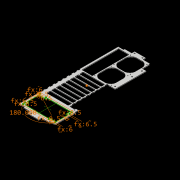
# Autodesk Inventor part: backpanel
Saved by Autodesk Inventor 2018 (Build 220112000, 112)
## iProperties
Created: 2019-10-14
Part Number: backpanel
Material: アルミニウム 6061
Document SubType Name: Modeling
Designer: gisen
Density: 2.7 g/cm^3
Appearance: アルミニウム - フラット
Author: gisen
Autodesk Inventor part; units mm, degrees
ref_plane "YZ Plane" through (0, 0, 0) normal (1, 0, 0) x (0, 1, 0)
ref_plane "XZ Plane" through (0, 0, 0) normal (0, 1, 0) x (-1, 0, 0)
ref_plane "XY Plane" through (0, 0, 0) normal (0, 0, 1) x (1, 0, 0)
sketch "スケッチ1" plane through (0, 0, 0) normal (0, 0, 1) x (1, 0, 0)
  line L0 (-55, -215) -> (55, -215) construction
  line L1 (55, -215) -> (55, 215) construction
  line L2 (55, 215) -> (-55, 215) construction
  line L3 (-55, 215) -> (-55, -215) construction
  line L4 (-55, -215) -> (55, 215) construction
  line L5 (55, -215) -> (-55, 215) construction
  line L6 (-75, 215) -> (-55, 215)
  line L7 (-55, 215) -> (-55, 232.5)
  line L8 (-55, 232.5) -> (55, 232.5)
  line L9 (55, 232.5) -> (55, 215)
  line L10 (55, 215) -> (75, 215)
  line L11 (75, 215) -> (75, -215)
  line L12 (75, -215) -> (55, -215)
  line L13 (55, -215) -> (55, -232.5)
  line L14 (55, -232.5) -> (-55, -232.5)
  line L15 (-55, -232.5) -> (-55, -215)
  line L16 (-55, -215) -> (-75, -215)
  line L17 (-75, -215) -> (-75, 215)
  line L18 (-65, 225) -> (65, 225) construction
  line L19 (65, 225) -> (65, -225) construction
  line L20 (65, -225) -> (-65, -225) construction
  line L21 (-65, -225) -> (-65, 225) construction
  circle A0 centre (-45, 225) radius 2.25
  circle A1 centre (-65, 205) radius 2.25
  line L22 (0, 0) -> (0, 232.5) construction
  line L23 (0, 0) -> (-75, 0) construction
  circle A2 centre (45, 225) radius 2.25
  circle A3 centre (65, 205) radius 2.25
  circle A4 centre (-45, -225) radius 2.25
  circle A5 centre (-65, -205) radius 2.25
  circle A6 centre (45, -225) radius 2.25
  circle A7 centre (65, -205) radius 2.25
  dimension "d0" = 110
  dimension "d1" = 430
  dimension "d2" = 17.5
  dimension "d3" = 17.5
  dimension "d4" = 20
  dimension "d5" = 20
  dimension "d6" = 10
  dimension "d7" = 10
  dimension "d8" = 10
  dimension "d9" = 10
  dimension "d10" = 4.5
  dimension "d11" = 10
  dimension "d12" = 10
  constraints: 48 end point, 8 centre point, 6 perpendicular, 6 point on line, 6 symmetric about line, 5 parallel, 4 midpoint, 4 vertical, 3 horizontal, 1 equal radius, 6 other
  measures "d0" distance of L2.end L1.end
  measures "d1" distance of L1.end L0.end
  measures "d2" distance of L8.end L1.end
  measures "d3" distance of L0.end L13.end
  measures "d4" distance of L1.end L10.end
  measures "d5" distance of L6.start L2.end
  measures "d6" distance between parallel lines of L2 L18
  measures "d7" distance between parallel lines of L3 L21
  measures "d8" distance between parallel lines of L0 L20
  measures "d9" distance between parallel lines of L1 L19
  measures "d10" diameter of A0
  measures "d11" distance from line of L7 A0.centre
  measures "d12" distance from line of A1.centre L6
extrude "押し出し1" add sketch "スケッチ1" along normal blind 3 contours L6 L7 L8 L9 L10 L11 L12 L13 L14 L15 L16 L17 | A1 | A5 | A7
sketch "スケッチ2" plane through (0, 0, 3) normal (0, 0, 1) x (1, 0, 0)
  line L0 (-68.0594, 208.0035) -> (-25.8794, 208.0035) construction
  line L1 (-69.2594, 50.3235) -> (-69.2594, 206.8035) construction
  line L2 (-25.8794, 49.1235) -> (-68.0594, 49.1235) construction
  line L3 (-24.6794, 206.8035) -> (-24.6794, 50.3235) construction
  line L4 (-24.6794, 49.1235) -> (-69.2594, 49.1235) construction
  line L5 (-69.2594, 49.1235) -> (-69.2594, 208.0035) construction
  line L6 (-69.2594, 208.0035) -> (-24.6794, 208.0035) construction
  line L7 (-24.6794, 208.0035) -> (-24.6794, 49.1235) construction
  line L8 (-24.6794, 49.1235) -> (-69.2594, 208.0035) construction
  line L9 (-69.2594, 49.1235) -> (-24.6794, 208.0035) construction
  line L10 (-69.3194, 49.0635) -> (-24.6194, 49.0635)
  line L11 (-24.6194, 49.0635) -> (-24.6194, 208.0635)
  line L12 (-24.6194, 208.0635) -> (-69.3194, 208.0635)
  line L13 (-69.3194, 208.0635) -> (-69.3194, 49.0635)
  line L14 (-69.3194, 49.0635) -> (-24.6194, 208.0635) construction
  line L15 (-24.6194, 49.0635) -> (-69.3194, 208.0635) construction
  point P0 (0, 0)
  point P1 (-46.9694, 128.5635)
  point P2 (-46.9694, 208.0035)
  point P3 (-69.2594, 128.5635)
  dimension "d16" = 44.7
  dimension "d17" = 159
  constraints: 24 end point, 8 midpoint, 4 parallel, 2 horizontal, 2 perpendicular
  measures "d16" distance of L12.end L11.end
  measures "d17" distance of L11.end L10.end
extrude "押し出し2" cut sketch "スケッチ2" against normal blind 3
sketch "スケッチ3" plane through (0, 0, 3) normal (0, 0, 1) x (1, 0, 0)
  line L0 (-70.0884, -112.7392) -> (-77.313, -112.7392) construction
  line L1 (-77.313, -102.4522) -> (-70.0884, -102.4522) construction
  line L2 (-70.0884, -92.3938) -> (-77.313, -92.3938) construction
  line L3 (-77.313, -82.1068) -> (-70.0884, -82.1068) construction
  line L4 (-70.0884, -71.7392) -> (-77.313, -71.7392) construction
  line L5 (-77.313, -61.4522) -> (-70.0884, -61.4522) construction
  line L6 (-70.0884, -51.3938) -> (-77.313, -51.3938) construction
  line L7 (-77.313, -41.1068) -> (-70.0884, -41.1068) construction
  line L8 (-70.0884, -30.7392) -> (-77.313, -30.7392) construction
  line L9 (-77.313, -20.4522) -> (-70.0884, -20.4522) construction
  line L10 (-70.0884, -10.3938) -> (-77.313, -10.3938) construction
  line L11 (-77.313, -0.1068) -> (-70.0884, -0.1068) construction
  line L12 (-70.0884, 10.2608) -> (-77.313, 10.2608) construction
  line L13 (-77.313, 20.5478) -> (-70.0884, 20.5478) construction
  line L14 (-70.0884, 30.6062) -> (-77.313, 30.6062) construction
  line L15 (-77.313, 40.8932) -> (-70.0884, 40.8932) construction
  line L16 (-75, 215) -> (-75, -215) projected
  line L17 (-75, 46.0635) -> (-78, 46.0635)
  line L18 (-78, 46.0635) -> (-78, 215)
  line L19 (-78, 215) -> (-75, 215)
  line L20 (-75, 215) -> (-75, 46.0635)
  line L21 (-24.6194, 49.0635) -> (-69.3194, 49.0635) projected
  line L22 (-75, -112.7392) -> (-78, -112.7392)
  line L23 (-78, -112.7392) -> (-78, -102.4522)
  line L24 (-78, -102.4522) -> (-75, -102.4522)
  line L25 (-75, -102.4522) -> (-75, -112.7392)
  line L26 (-75, -92.3938) -> (-78, -92.3938)
  line L27 (-78, -92.3938) -> (-78, -82.1068)
  line L28 (-78, -82.1068) -> (-75, -82.1068)
  line L29 (-75, -82.1068) -> (-75, -92.3938)
  line L30 (-75, -71.7392) -> (-78, -71.7392)
  line L31 (-78, -71.7392) -> (-78, -61.4522)
  line L32 (-78, -61.4522) -> (-75, -61.4522)
  line L33 (-75, -61.4522) -> (-75, -71.7392)
  line L34 (-75, -51.3938) -> (-78, -51.3938)
  line L35 (-78, -51.3938) -> (-78, -41.1068)
  line L36 (-78, -41.1068) -> (-75, -41.1068)
  line L37 (-75, -41.1068) -> (-75, -51.3938)
  line L38 (-75, -30.7392) -> (-78, -30.7392)
  line L39 (-78, -30.7392) -> (-78, -20.4522)
  line L40 (-78, -20.4522) -> (-75, -20.4522)
  line L41 (-75, -20.4522) -> (-75, -30.7392)
  line L42 (-75, -10.3938) -> (-78, -10.3938)
  line L43 (-78, -10.3938) -> (-78, -0.1068)
  line L44 (-78, -0.1068) -> (-75, -0.1068)
  line L45 (-75, -0.1068) -> (-75, -10.3938)
  line L46 (-75, 10.2608) -> (-78, 10.2608)
  line L47 (-78, 10.2608) -> (-78, 20.5478)
  line L48 (-78, 20.5478) -> (-75, 20.5478)
  line L49 (-75, 20.5478) -> (-75, 10.2608)
  line L50 (-75, 30.6062) -> (-78, 30.6062)
  line L51 (-78, 30.6062) -> (-78, 40.8932)
  line L52 (-78, 40.8932) -> (-75, 40.8932)
  line L53 (-75, 40.8932) -> (-75, 30.6062)
  point P0 (0, 0)
  dimension "d20" = 3
  dimension "d21" = 3
  constraints: 72 end point, 26 parallel, 16 point on line, 9 horizontal, 9 perpendicular, 10 other
  measures "d20" distance of L19.end L18.end
  measures "d21" distance between parallel lines of L21 L17
extrude "押し出し3" add sketch "スケッチ3" against normal blind 3
sketch "スケッチ4" plane through (0, 0, 3) normal (0, 0, 1) x (1, 0, 0)
  line L0 (-67.0004, 201.5535) -> (-67.0004, -95.6265) construction
  line L1 (-78, 40.8932) -> (-78, 30.6062) construction
  line L2 (-78, 20.5478) -> (-78, 10.2608) construction
  line L3 (-78, -0.1068) -> (-78, -10.3938) construction
  line L4 (-78, -20.4522) -> (-78, -30.7392) construction
  line L5 (-78, -41.1068) -> (-78, -51.3938) construction
  line L6 (-78, -61.4522) -> (-78, -71.7392) construction
  line L7 (-78, -82.1068) -> (-78, -92.3938) construction
  line L8 (-78, -102.4522) -> (-78, -112.7392) construction
  line L9 (-78, 35.7497) -> (-12.1004, 35.7497) construction
  line L10 (-58.9404, 27.8097) -> (34.7396, 27.8097)
  line L11 (34.7396, 27.8097) -> (34.7396, 43.6897) construction
  line L12 (34.7396, 43.6897) -> (-58.9404, 43.6897)
  line L13 (-58.9404, 43.6897) -> (-58.9404, 27.8097)
  line L14 (-58.9404, 27.8097) -> (34.7396, 43.6897) construction
  line L15 (34.7396, 27.8097) -> (-58.9404, 43.6897) construction
  line L16 (34.7396, 43.6897) -> (34.7396, 40.5147)
  line L17 (34.7396, 40.5147) -> (35.0196, 40.5147)
  line L18 (35.0196, 40.5147) -> (35.0196, 30.9847)
  line L19 (35.0196, 30.9847) -> (34.7396, 30.9847)
  line L20 (34.7396, 30.9847) -> (34.7396, 27.8097)
  line L21 (42.7196, 40.3787) -> (42.7196, 47.7987) construction
  line L22 (-75, 20.5478) -> (-78, 20.5478) construction
  line L23 (-75, 40.8932) -> (-78, 40.8932) construction
  line L24 (-58.9404, 7.4643) -> (34.7396, 7.4643)
  line L25 (-58.9404, 23.3443) -> (-58.9404, 7.4643)
  line L26 (34.7396, 23.3443) -> (-58.9404, 23.3443)
  line L27 (34.7396, 23.3443) -> (34.7396, 20.1693)
  line L28 (34.7396, 20.1693) -> (35.0196, 20.1693)
  line L29 (35.0196, 20.1693) -> (35.0196, 10.6393)
  line L30 (35.0196, 10.6393) -> (34.7396, 10.6393)
  line L31 (34.7396, 10.6393) -> (34.7396, 7.4643)
  line L32 (-58.9404, -12.8811) -> (34.7396, -12.8811)
  line L33 (-58.9404, 2.9989) -> (-58.9404, -12.8811)
  line L34 (34.7396, 2.9989) -> (-58.9404, 2.9989)
  line L35 (34.7396, 2.9989) -> (34.7396, -0.1761)
  line L36 (34.7396, -0.1761) -> (35.0196, -0.1761)
  line L37 (35.0196, -0.1761) -> (35.0196, -9.7061)
  line L38 (35.0196, -9.7061) -> (34.7396, -9.7061)
  line L39 (34.7396, -9.7061) -> (34.7396, -12.8811)
  line L40 (-58.9404, -33.2265) -> (34.7396, -33.2265)
  line L41 (-58.9404, -17.3465) -> (-58.9404, -33.2265)
  line L42 (34.7396, -17.3465) -> (-58.9404, -17.3465)
  line L43 (34.7396, -17.3465) -> (34.7396, -20.5215)
  line L44 (34.7396, -20.5215) -> (35.0196, -20.5215)
  line L45 (35.0196, -20.5215) -> (35.0196, -30.0515)
  line L46 (35.0196, -30.0515) -> (34.7396, -30.0515)
  line L47 (34.7396, -30.0515) -> (34.7396, -33.2265)
  line L48 (-58.9404, -53.5719) -> (34.7396, -53.5719)
  line L49 (-58.9404, -37.6919) -> (-58.9404, -53.5719)
  line L50 (34.7396, -37.6919) -> (-58.9404, -37.6919)
  line L51 (34.7396, -37.6919) -> (34.7396, -40.8669)
  line L52 (34.7396, -40.8669) -> (35.0196, -40.8669)
  line L53 (35.0196, -40.8669) -> (35.0196, -50.3969)
  line L54 (35.0196, -50.3969) -> (34.7396, -50.3969)
  line L55 (34.7396, -50.3969) -> (34.7396, -53.5719)
  line L56 (-58.9404, -73.9173) -> (34.7396, -73.9173)
  line L57 (-58.9404, -58.0373) -> (-58.9404, -73.9173)
  line L58 (34.7396, -58.0373) -> (-58.9404, -58.0373)
  line L59 (34.7396, -58.0373) -> (34.7396, -61.2123)
  line L60 (34.7396, -61.2123) -> (35.0196, -61.2123)
  line L61 (35.0196, -61.2123) -> (35.0196, -70.7423)
  line L62 (35.0196, -70.7423) -> (34.7396, -70.7423)
  line L63 (34.7396, -70.7423) -> (34.7396, -73.9173)
  line L64 (-58.9404, -94.2627) -> (34.7396, -94.2627)
  line L65 (-58.9404, -78.3827) -> (-58.9404, -94.2627)
  line L66 (34.7396, -78.3827) -> (-58.9404, -78.3827)
  line L67 (34.7396, -78.3827) -> (34.7396, -81.5577)
  line L68 (34.7396, -81.5577) -> (35.0196, -81.5577)
  line L69 (35.0196, -81.5577) -> (35.0196, -91.0877)
  line L70 (35.0196, -91.0877) -> (34.7396, -91.0877)
  line L71 (34.7396, -91.0877) -> (34.7396, -94.2627)
  line L72 (-58.9404, -114.6081) -> (34.7396, -114.6081)
  line L73 (-58.9404, -98.7281) -> (-58.9404, -114.6081)
  line L74 (34.7396, -98.7281) -> (-58.9404, -98.7281)
  line L75 (34.7396, -98.7281) -> (34.7396, -101.9031)
  line L76 (34.7396, -101.9031) -> (35.0196, -101.9031)
  line L77 (35.0196, -101.9031) -> (35.0196, -111.4331)
  line L78 (35.0196, -111.4331) -> (34.7396, -111.4331)
  line L79 (34.7396, -111.4331) -> (34.7396, -114.6081)
  line L80 (75, -215) -> (75, 215) projected
  line L81 (42.2196, -115.1237) -> (75, -115.1237)
  line L82 (75, -115.1237) -> (75, 48.3987)
  line L83 (75, 48.3987) -> (42.2196, 48.3987)
  line L84 (42.2196, 48.3987) -> (42.2196, -115.1237)
  line L85 (42.8196, 47.8987) -> (43.6196, 47.8987) projected
  line L86 (43.6196, -114.6237) -> (42.8196, -114.6237) construction
  point P0 (0, 0)
  point P1 (35.0196, 35.7497)
  point P2 (35.0196, 15.4043)
  point P3 (35.0196, -4.9411)
  point P4 (35.0196, -25.2865)
  point P5 (35.0196, -45.6319)
  point P6 (35.0196, -65.9773)
  point P7 (35.0196, -86.3227)
  point P8 (35.0196, -106.6681)
  dimension "d24" = 8.06
  dimension "d25" = 93.68
  dimension "d26" = 15.88
  dimension "d27" = 9.53
  dimension "d28" = 7.7
  dimension "d29" = 20.3454
  dimension "d32" = 20.3454
  dimension "d38" = 0.5
  dimension "d39" = 0.5
  dimension "d97" = 0.5
  constraints: 144 end point, 4 horizontal, 4 midpoint, 4 parallel, 4 perpendicular, 4 point on line, 1 collinear, 1 vertical, 119 other
  measures "d24" distance between parallel lines of L0 L13
  measures "d25" distance of L11.end L12.end
  measures "d26" distance of L12.end L10.start
  measures "d27" distance of L17.end L18.end
  measures "d28" distance between parallel lines of L18 L21
  measures "d29" distance between parallel lines of L22 L23
  measures "d32" distance of L10.start L24.start
  measures "d38" distance from line of L21 L83.end
  measures "d39" distance between parallel lines of L81 L86
  measures "d97" distance between parallel lines of L85 L83
extrude "押し出し4" cut sketch "スケッチ4" against normal blind 3
sketch "スケッチ5" plane through (0, 0, 3) normal (0, 0, 1) x (1, 0, 0)
  circle A0 centre (-70, -132.4) radius 1.25 construction
  circle A1 centre (-70, -196.4) radius 1.25 construction
  circle A2 centre (44, -206.4) radius 1.25 construction
  circle A3 centre (68, -132.4) radius 1.25 construction
  line L0 (75, -127.8) -> (75, -201.1029) construction
  line L1 (-73.8, -126.6) -> (73.8, -126.6) construction
  line L2 (-75, -127.8) -> (-75, -201.1029) construction
  line L3 (73, -212) -> (-73, -212) construction
  line L4 (0, -126.6) -> (0, -212) construction
  line L5 (-70, -132.4) -> (-70, -135.4) construction
  line L6 (-71.75, -132.4) -> (-71.75, -135.4)
  line L7 (-68.25, -135.4) -> (-68.25, -132.4)
  arc A4 (-68.25, -132.4) -> (-71.75, -132.4) centre (-70, -132.4) ccw
  arc A5 (-71.75, -135.4) -> (-68.25, -135.4) centre (-70, -135.4) ccw
  line L8 (-44, -132.2) -> (-44, -135.2) construction
  line L9 (-45.75, -132.2) -> (-45.75, -135.2)
  line L10 (-42.25, -135.2) -> (-42.25, -132.2)
  arc A6 (-42.25, -132.2) -> (-45.75, -132.2) centre (-44, -132.2) ccw
  arc A7 (-45.75, -135.2) -> (-42.25, -135.2) centre (-44, -135.2) ccw
  line L11 (-70, -196.4) -> (-70, -199.4) construction
  line L12 (-72, -196.4) -> (-72, -199.4)
  line L13 (-68, -199.4) -> (-68, -196.4)
  arc A8 (-68, -196.4) -> (-72, -196.4) centre (-70, -196.4) ccw
  arc A9 (-72, -199.4) -> (-68, -199.4) centre (-70, -199.4) ccw
  line L14 (-68, -206.2) -> (-68, -209.2) construction
  line L15 (-69.75, -206.2) -> (-69.75, -209.2)
  line L16 (-66.25, -209.2) -> (-66.25, -206.2)
  arc A10 (-66.25, -206.2) -> (-69.75, -206.2) centre (-68, -206.2) ccw
  arc A11 (-69.75, -209.2) -> (-66.25, -209.2) centre (-68, -209.2) ccw
  line L17 (68, -132.4) -> (68, -135.4) construction
  line L18 (66.25, -132.4) -> (66.25, -135.4)
  line L19 (69.75, -135.4) -> (69.75, -132.4)
  arc A12 (69.75, -132.4) -> (66.25, -132.4) centre (68, -132.4) ccw
  arc A13 (66.25, -135.4) -> (69.75, -135.4) centre (68, -135.4) ccw
  line L20 (70, -142.2) -> (70, -145.2) construction
  line L21 (68.25, -142.2) -> (68.25, -145.2)
  line L22 (71.75, -145.2) -> (71.75, -142.2)
  arc A14 (71.75, -142.2) -> (68.25, -142.2) centre (70, -142.2) ccw
  arc A15 (68.25, -145.2) -> (71.75, -145.2) centre (70, -145.2) ccw
  line L23 (70, -206.2) -> (70, -209.2) construction
  line L24 (68.25, -206.2) -> (68.25, -209.2)
  line L25 (71.75, -209.2) -> (71.75, -206.2)
  arc A16 (71.75, -206.2) -> (68.25, -206.2) centre (70, -206.2) ccw
  arc A17 (68.25, -209.2) -> (71.75, -209.2) centre (70, -209.2) ccw
  line L26 (44, -206.4) -> (44, -209.4) construction
  line L27 (42.25, -206.4) -> (42.25, -209.4)
  line L28 (45.75, -209.4) -> (45.75, -206.4)
  arc A18 (45.75, -206.4) -> (42.25, -206.4) centre (44, -206.4) ccw
  arc A19 (42.25, -209.4) -> (45.75, -209.4) centre (44, -209.4) ccw
  line L29 (-69, -139.4) -> (-37.5, -139.4)
  line L30 (-37.5, -139.4) -> (-37.5, -132.6)
  line L31 (-37.5, -132.6) -> (61.5, -132.6)
  line L32 (61.5, -132.6) -> (61.5, -151.7)
  line L33 (61.5, -151.7) -> (69, -151.7)
  line L34 (69, -151.7) -> (69, -202.4)
  line L35 (69, -202.4) -> (37.5, -202.4)
  line L36 (37.5, -202.4) -> (37.5, -206)
  line L37 (37.5, -206) -> (-61.5, -206)
  line L38 (-61.5, -206) -> (-61.5, -189.9)
  line L39 (-61.5, -189.9) -> (-69, -189.9)
  line L40 (-69, -189.9) -> (-69, -139.4)
  point P0 (0, 0)
  point P1 (0, -169.3)
  point P2 (-70, -133.9)
  point P3 (-44, -133.7)
  point P4 (-70, -197.9)
  point P5 (-68, -207.7)
  point P6 (68, -133.9)
  point P7 (70, -143.7)
  point P8 (70, -207.7)
  point P9 (44, -207.9)
  dimension "d44" = 180
  dimension "d46" = 3.5
  dimension "d47" = 3
  dimension "d48" = 6
  dimension "d49" = 6
  dimension "d50" = 4
  dimension "d51" = 6.5
  dimension "d52" = 6.5
  dimension "d53" = 6.5
  dimension "d54" = 6
  dimension "d55" = 4
  dimension "d56" = 6.5
  dimension "d57" = 6
  dimension "d58" = 6.5
  dimension "d59" = 6.5
  constraints: 90 end point, 32 point on circle, 32 tangent, 16 centre point, 12 perpendicular, 11 midpoint, 11 parallel, 7 equal length, 6 equal radius, 4 vertical, 1 horizontal, 1 point on line, 5 other
  measures "d46" diameter of A5
  measures "d47" distance of L7.start L7.end
  measures "d48" distance between parallel lines of L2 L40
  measures "d49" distance between parallel lines of L0 L34
  measures "d50" distance from line of L29 L5.end
  measures "d51" distance from line of L8.end L30
  measures "d52" distance from line of L17.end L32
  measures "d53" distance from line of L33 L20.end
  measures "d54" distance between parallel lines of L31 L1
  measures "d55" distance from line of L26.start L35
  measures "d56" distance from line of L26.start L36
  measures "d57" distance between parallel lines of L3 L37
  measures "d58" distance from line of L14.start L38
  measures "d59" distance from line of L39 L11.start
extrude "押し出し5" cut sketch "スケッチ5" against normal blind 3
fillet "フィレット1" radius 3 12 edges at (69, -151.7, 1.5) (61.5, -151.7, 1.5) (61.5, -132.6, 1.5) (-37.5, -132.6, 1.5) (-37.5, -139.4, 1.5) (-69, -139.4, 1.5) (-69, -189.9, 1.5) (-61.5, -189.9, 1.5) (-61.5, -206, 1.5) (37.5, -206, 1.5) (37.5, -202.4, 1.5) (69, -202.4, 1.5)
sketch "スケッチ6" plane through (0, 0, 3) normal (0, 0, 1) x (1, 0, 0)
  line L0 (-75, -215) -> (-55, -215) projected
  line L1 (-75, -215) -> (-78, -215)
  line L2 (-78, -215) -> (-78, -124.6)
  line L3 (-78, -124.6) -> (-75, -124.6)
  line L4 (-75, -124.6) -> (-75, -215)
  line L5 (-78, -112.7392) -> (-75, -112.7392) projected
  line L6 (-34.5, -132.6) -> (58.5, -132.6) projected
  point P0 (0, 0)
  dimension "d63" = 8
  constraints: 8 end point, 3 parallel, 1 horizontal, 1 perpendicular
  measures "d63" distance between parallel lines of L6 L3
extrude "押し出し6" add sketch "スケッチ6" against normal blind 3
sketch "スケッチ7" plane through (0, 0, 3) normal (0, 0, 1) x (1, 0, 0)
  line L0 (56.3806, 130.3987) -> (-23.6194, 130.3987) construction
  line L1 (-23.6194, 130.3987) -> (-23.6194, 50.3987) construction
  line L2 (-23.6194, 50.3987) -> (56.3806, 50.3987) construction
  line L3 (56.3806, 50.3987) -> (56.3806, 130.3987) construction
  line L4 (56.3806, 130.3987) -> (-23.6194, 50.3987) construction
  line L5 (-23.6194, 130.3987) -> (56.3806, 50.3987) construction
  line L6 (-23.6194, 213.3987) -> (56.3806, 213.3987) construction
  line L7 (56.3806, 213.3987) -> (56.3806, 133.3987) construction
  line L8 (56.3806, 133.3987) -> (-23.6194, 133.3987) construction
  line L9 (-23.6194, 133.3987) -> (-23.6194, 213.3987) construction
  line L10 (-23.6194, 213.3987) -> (56.3806, 133.3987) construction
  line L11 (56.3806, 213.3987) -> (-23.6194, 133.3987) construction
  line L12 (42.2196, 48.3987) -> (75, 48.3987) construction
  line L13 (-24.6194, 208.0635) -> (-24.6194, 49.0635) construction
  circle A0 centre (16.3806, 90.3987) radius 42.5 construction
  line L14 (-22.4194, 51.5987) -> (55.1806, 51.5987) construction
  line L15 (55.1806, 51.5987) -> (55.1806, 129.1987) construction
  line L16 (55.1806, 129.1987) -> (-22.4194, 129.1987) construction
  line L17 (-22.4194, 129.1987) -> (-22.4194, 51.5987) construction
  line L18 (-22.4194, 51.5987) -> (55.1806, 129.1987) construction
  line L19 (55.1806, 51.5987) -> (-22.4194, 129.1987) construction
  line L20 (-19.3694, 54.6487) -> (52.1306, 54.6487) construction
  line L21 (52.1306, 54.6487) -> (52.1306, 126.1487) construction
  line L22 (52.1306, 126.1487) -> (-19.3694, 126.1487) construction
  line L23 (-19.3694, 126.1487) -> (-19.3694, 54.6487) construction
  line L24 (-19.3694, 54.6487) -> (52.1306, 126.1487) construction
  line L25 (52.1306, 54.6487) -> (-19.3694, 126.1487) construction
  arc A1 (-0.9633, 129.1987) -> (-22.4194, 107.7426) centre (16.3806, 90.3987) ccw
  arc A2 (55.1806, 107.7426) -> (33.7245, 129.1987) centre (16.3806, 90.3987) ccw
  arc A3 (-22.4194, 73.0549) -> (-0.9633, 51.5987) centre (16.3806, 90.3987) ccw
  arc A4 (33.7245, 51.5987) -> (55.1806, 73.0549) centre (16.3806, 90.3987) ccw
  line L26 (-22.4194, 107.7426) -> (-22.4194, 73.0549)
  line L27 (-0.9633, 51.5987) -> (33.7245, 51.5987)
  line L28 (55.1806, 107.7426) -> (55.1806, 73.0549)
  line L29 (-0.9633, 129.1987) -> (33.7245, 129.1987)
  circle A5 centre (-19.3694, 126.1487) radius 1.2
  circle A6 centre (52.1306, 126.1487) radius 1.2
  circle A7 centre (-19.3694, 54.6487) radius 1.2
  circle A8 centre (52.1306, 54.6487) radius 1.2
  circle A9 centre (-19.3694, 209.1487) radius 1.2
  arc A10 (-0.9633, 212.1987) -> (-22.4194, 190.7426) centre (16.3806, 173.3987) ccw
  line L30 (-0.9633, 212.1987) -> (33.7245, 212.1987)
  arc A11 (55.1806, 190.7426) -> (33.7245, 212.1987) centre (16.3806, 173.3987) ccw
  circle A12 centre (52.1306, 209.1487) radius 1.2
  line L31 (55.1806, 190.7426) -> (55.1806, 156.0549)
  arc A13 (33.7245, 134.5987) -> (55.1806, 156.0549) centre (16.3806, 173.3987) ccw
  line L32 (-0.9633, 134.5987) -> (33.7245, 134.5987)
  circle A14 centre (52.1306, 137.6487) radius 1.2
  circle A15 centre (-19.3694, 137.6487) radius 1.2
  arc A16 (-22.4194, 156.0549) -> (-0.9633, 134.5987) centre (16.3806, 173.3987) ccw
  line L33 (-22.4194, 190.7426) -> (-22.4194, 156.0549)
  point P0 (0, 0)
  point P1 (16.3806, 173.3987)
  dimension "d74" = 85
  dimension "d66" = 80
  dimension "d67" = 80
  dimension "d68" = 80
  dimension "d69" = 80
  dimension "d70" = 3
  dimension "d71" = 2
  dimension "d73" = 1
  dimension "d78" = 71.5
  dimension "d79" = 71.5
  dimension "d80" = 2.4
  dimension "d81" = 77.6
  dimension "d84" = 83
  constraints: 64 end point, 16 centre point, 16 point on circle, 12 midpoint, 10 coincident, 9 parallel, 9 point on line, 6 perpendicular, 4 horizontal, 3 equal radius, 1 collinear, 1 vertical, 38 other
  measures "d66" distance of L2.end L1.end
  measures "d67" distance of L1.end L0.end
  measures "d68" distance of L7.end L8.end
  measures "d69" distance of L6.end L7.end
  measures "d70" distance between parallel lines of L0 L8
  measures "d71" distance between parallel lines of L12 L2
  measures "d73" distance between parallel lines of L13 L9
  measures "d78" distance of L22.end L21.end
  measures "d79" distance of L21.end L20.end
  measures "d80" diameter of A5
  measures "d81" distance of L15.end L16.end
  measures "d84" distance of A5.centre A9.centre
extrude "押し出し7" cut sketch "スケッチ7" against normal blind 3
sketch "スケッチ8" plane through (0, 0, 3) normal (0, 0, 1) x (1, 0, 0)
  arc A0 (-0.9633, 129.1987) -> (-22.4194, 107.7426) centre (16.3806, 90.3987) ccw projected
  line L0 (-19.6194, 112.9875) -> (-22.4194, 112.9875)
  line L1 (-22.4194, 112.9875) -> (-22.4194, 67.81)
  line L2 (-22.4194, 67.81) -> (-19.6194, 67.81)
  line L3 (-19.6194, 67.81) -> (-19.6194, 112.9875)
  arc A1 (-22.4194, 73.0549) -> (-0.9633, 51.5987) centre (16.3806, 90.3987) ccw projected
  line L4 (-22.4194, 73.0549) -> (-22.4194, 107.7426) projected
  arc A2 (-22.4194, 156.0549) -> (-0.9633, 134.5987) centre (16.3806, 173.3987) ccw projected
  line L5 (-19.6194, 150.81) -> (-22.4194, 150.81)
  line L6 (-22.4194, 150.81) -> (-22.4194, 195.9875)
  line L7 (-22.4194, 195.9875) -> (-19.6194, 195.9875)
  line L8 (-19.6194, 195.9875) -> (-19.6194, 150.81)
  arc A3 (-0.9633, 212.1987) -> (-22.4194, 190.7426) centre (16.3806, 173.3987) ccw projected
  line L9 (-22.4194, 156.0549) -> (-22.4194, 190.7426) projected
  line L10 (16.3806, 173.3987) -> (16.3806, 90.3987) construction
  line L11 (52.3806, 112.9875) -> (55.1806, 112.9875)
  line L12 (55.1806, 112.9875) -> (55.1806, 67.81)
  line L13 (55.1806, 67.81) -> (52.3806, 67.81)
  line L14 (52.3806, 67.81) -> (52.3806, 112.9875)
  line L15 (55.1806, 73.0549) -> (55.1806, 107.7426)
  line L16 (52.3806, 150.81) -> (55.1806, 150.81)
  line L17 (55.1806, 150.81) -> (55.1806, 195.9875)
  line L18 (55.1806, 195.9875) -> (52.3806, 195.9875)
  line L19 (52.3806, 195.9875) -> (52.3806, 150.81)
  line L20 (55.1806, 156.0549) -> (55.1806, 190.7426)
  point P0 (0, 0)
  dimension "d92" = 2.8
  constraints: 38 end point, 12 symmetric about line, 5 parallel, 4 point on circle, 4 point on line, 2 horizontal, 2 perpendicular, 1 vertical
  measures "d92" distance between parallel lines of L1 L3
extrude "押し出し8" add sketch "スケッチ8" against normal blind 3 contours L3 A1 L1 A0 | L6 A3 L8 A2 | L11 L12 L13 L14 | L19 L18 L17 L16
fillet "フィレット3" radius 3 32 edges at (-58.9404, 43.6897, 1.5) (-58.9404, 27.8097, 1.5) (-58.9404, 23.3443, 1.5) (-58.9404, 7.4643, 1.5) (-58.9404, 2.9989, 1.5) (-58.9404, -12.8811, 1.5) (-58.9404, -17.3465, 1.5) (-58.9404, -33.2265, 1.5) (-58.9404, -37.6919, 1.5) (-58.9404, -53.5719, 1.5) (-58.9404, -58.0373, 1.5) (-58.9404, -73.9173, 1.5) (-58.9404, -78.3827, 1.5) (-58.9404, -94.2627, 1.5) (-58.9404, -98.7281, 1.5) (-58.9404, -114.6081, 1.5) (34.7396, 43.6897, 1.5) (34.7396, 27.8097, 1.5) (34.7396, 23.3443, 1.5) (34.7396, -12.8811, 1.5) (34.7396, -17.3465, 1.5) (34.7396, -33.2265, 1.5) (34.7396, -37.6919, 1.5) (34.7396, -53.5719, 1.5) (34.7396, -58.0373, 1.5) (34.7396, -73.9173, 1.5) (34.7396, -78.3827, 1.5) (34.7396, -94.2627, 1.5) (34.7396, -98.7281, 1.5) (34.7396, -114.6081, 1.5) (34.7396, 7.4643, 1.5) (34.7396, 2.9989, 1.5)
sketch "スケッチ9" plane through (0, 0, 3) normal (0, 0, 1) x (1, 0, 0)
  line L0 (42.8196, -15.4787) -> (42.8196, -16.9804) construction
  line L1 (42.8196, -16.9813) -> (42.8196, -19.1617) construction
  line L2 (42.8196, -13.3198) -> (42.8196, -15.4787) construction
  line L3 (43.6196, 1.4123) -> (43.6196, 3.5713) construction
  line L4 (43.6196, 6.7987) -> (43.6196, 3.5713) construction
  line L5 (43.6196, 21.8383) -> (43.6196, 24.0187) construction
  line L6 (43.6196, 25.5213) -> (43.6196, 24.0196) construction
  line L7 (43.6196, 25.5213) -> (43.6196, 27.6802) construction
  line L8 (43.6196, 42.4123) -> (43.6196, 44.5713) construction
  line L9 (43.6196, 47.7987) -> (43.6196, 44.5713) construction
  line L10 (43.6196, 24.7705) -> (39.1196, 24.7705) construction
  line L11 (43.6196, -16.9804) -> (43.6196, -15.4787) construction
  line L12 (42.8196, -16.2295) -> (39.1196, -16.2295) construction
  line L13 (39.1196, 24.7705) -> (39.1196, -16.2295) construction
  line L14 (39.1196, 24.7705) -> (39.1196, 45.2705) construction
  line L15 (39.1196, 45.2705) -> (40.6696, 45.2705) construction
  line L16 (42.2196, -115.1237) -> (42.2196, 48.3987) projected
  line L17 (39.1196, 42.2705) -> (42.2196, 42.2705)
  line L18 (42.2196, 42.2705) -> (42.2196, 48.2705)
  line L19 (42.2196, 48.2705) -> (39.1196, 48.2705)
  line L20 (39.1196, 48.2705) -> (39.1196, 42.2705)
  line L21 (39.1196, 42.2705) -> (42.2196, 48.2705) construction
  line L22 (42.2196, 42.2705) -> (39.1196, 48.2705) construction
  line L23 (42.2196, 21.7705) -> (39.1196, 21.7705)
  line L24 (39.1196, 21.7705) -> (39.1196, 27.7705)
  line L25 (39.1196, 27.7705) -> (42.2196, 27.7705)
  line L26 (42.2196, 27.7705) -> (42.2196, 21.7705)
  line L27 (42.2196, 21.7705) -> (39.1196, 27.7705) construction
  line L28 (39.1196, 21.7705) -> (42.2196, 27.7705) construction
  line L29 (42.2196, 7.2705) -> (39.1196, 7.2705)
  line L30 (39.1196, 4.2705) -> (40.6696, 4.2705) construction
  line L31 (42.2196, 1.2705) -> (42.2196, 7.2705)
  line L32 (39.1196, 7.2705) -> (39.1196, 1.2705)
  line L33 (39.1196, 1.2705) -> (42.2196, 7.2705) construction
  line L34 (39.1196, 1.2705) -> (42.2196, 1.2705)
  line L35 (42.2196, 1.2705) -> (39.1196, 7.2705) construction
  line L36 (42.2196, -19.2295) -> (39.1196, -19.2295)
  line L37 (42.2196, -13.2295) -> (42.2196, -19.2295)
  line L38 (39.1196, -19.2295) -> (39.1196, -13.2295)
  line L39 (42.2196, -19.2295) -> (39.1196, -13.2295) construction
  line L40 (39.1196, -19.2295) -> (42.2196, -13.2295) construction
  line L41 (39.1196, -13.2295) -> (42.2196, -13.2295)
  line L42 (43.6196, -16.2295) -> (39.1196, -16.2295) construction
  line L43 (42.2196, -33.7295) -> (39.1196, -33.7295)
  line L44 (39.1196, -36.7295) -> (40.6696, -36.7295) construction
  line L45 (42.2196, -39.7295) -> (42.2196, -33.7295)
  line L46 (39.1196, -33.7295) -> (39.1196, -39.7295)
  line L47 (39.1196, -39.7295) -> (42.2196, -33.7295) construction
  line L48 (39.1196, -39.7295) -> (42.2196, -39.7295)
  line L49 (42.2196, -39.7295) -> (39.1196, -33.7295) construction
  line L50 (42.2196, -60.2295) -> (39.1196, -60.2295)
  line L51 (42.2196, -54.2295) -> (42.2196, -60.2295)
  line L52 (39.1196, -60.2295) -> (39.1196, -54.2295)
  line L53 (42.2196, -60.2295) -> (39.1196, -54.2295) construction
  line L54 (39.1196, -60.2295) -> (42.2196, -54.2295) construction
  line L55 (39.1196, -54.2295) -> (42.2196, -54.2295)
  line L56 (43.6196, -57.2295) -> (39.1196, -57.2295) construction
  line L57 (42.2196, -74.7295) -> (39.1196, -74.7295)
  line L58 (39.1196, -77.7295) -> (40.6696, -77.7295) construction
  line L59 (42.2196, -80.7295) -> (42.2196, -74.7295)
  line L60 (39.1196, -74.7295) -> (39.1196, -80.7295)
  line L61 (39.1196, -80.7295) -> (42.2196, -74.7295) construction
  line L62 (39.1196, -80.7295) -> (42.2196, -80.7295)
  line L63 (42.2196, -80.7295) -> (39.1196, -74.7295) construction
  line L64 (42.2196, -101.2295) -> (39.1196, -101.2295)
  line L65 (42.2196, -95.2295) -> (42.2196, -101.2295)
  line L66 (39.1196, -101.2295) -> (39.1196, -95.2295)
  line L67 (42.2196, -101.2295) -> (39.1196, -95.2295) construction
  line L68 (39.1196, -101.2295) -> (42.2196, -95.2295) construction
  line L69 (39.1196, -95.2295) -> (42.2196, -95.2295)
  line L70 (43.6196, -98.2295) -> (39.1196, -98.2295) construction
  point P0 (0, 0)
  point P1 (40.6696, 24.7705)
  point P2 (43.6196, 1.4123)
  point P3 (43.6196, 3.5713)
  point P4 (43.6196, 6.7987)
  point P5 (42.2196, 7.3987)
  point P6 (43.6196, -16.9804)
  point P7 (40.6696, -16.2295)
  point P8 (43.6196, -16.9813)
  point P9 (43.6196, -15.4787)
  point P10 (43.6196, -13.3198)
  point P11 (43.6196, -19.1617)
  point P12 (43.6196, -39.5877)
  point P13 (43.6196, -37.4287)
  point P14 (43.6196, -34.2013)
  point P15 (42.2196, -33.6013)
  point P16 (43.6196, -57.9804)
  point P17 (40.6696, -57.2295)
  point P18 (43.6196, -57.9813)
  point P19 (43.6196, -56.4787)
  point P20 (43.6196, -54.3198)
  point P21 (43.6196, -60.1617)
  point P22 (43.6196, -80.5877)
  point P23 (43.6196, -78.4287)
  point P24 (43.6196, -75.2013)
  point P25 (42.2196, -74.6013)
  point P26 (43.6196, -98.9804)
  point P27 (40.6696, -98.2295)
  point P28 (43.6196, -98.9813)
  point P29 (43.6196, -97.4787)
  point P30 (43.6196, -95.3198)
  point P31 (43.6196, -101.1617)
  dimension "d98" = 4.5
  dimension "d99" = 0.6992
  dimension "d100" = 0.7518
  dimension "d101" = 41
  dimension "d102" = 6
  dimension "d105" = 41
  dimension "d154" = 41
  dimension "d155" = 20.5
  constraints: 118 end point, 18 midpoint, 8 point on line, 5 horizontal, 4 parallel, 3 vertical, 2 perpendicular, 1 collinear, 108 other
  measures "d98" distance of L10.start L10.end
  measures "d99" vertical distance of L8.end L14.end
  measures "d100" distance from line of L5.end L10
  measures "d101" distance from line of L12.end L10
  measures "d102" distance of L19.end L17.start
  measures "d105" distance of L8.start point (43.62, 1.412)
  measures "d154" distance from line of point (40.67, -16.23) L10
  measures "d155" distance of L15.end point (40.67, 24.77)
extrude "押し出し9" cut sketch "スケッチ9" against normal blind 3
sketch "スケッチ10" plane through (0, 0, 3) normal (0, 0, 1) x (1, 0, 0)
  line L0 (42.2196, -102.7295) -> (40.7196, -102.7295)
  line L1 (40.7196, -102.7295) -> (40.7196, 49.7705)
  line L2 (40.7196, 49.7705) -> (42.2196, 49.7705)
  line L3 (42.2196, 49.7705) -> (42.2196, -102.7295)
  line L4 (39.1196, 48.2705) -> (42.2196, 48.2705) projected
  line L5 (42.2196, -101.2295) -> (39.1196, -101.2295) projected
  line L6 (42.2196, -115.1237) -> (42.2196, -101.2295) projected
  point P0 (0, 0)
  dimension "d112" = 1.5
  dimension "d149" = 1.5
  dimension "d150" = 1.5
  constraints: 8 end point, 2 parallel, 1 horizontal, 1 perpendicular, 1 point on line
  measures "d112" distance of L0.start L0.end
  measures "d149" distance between parallel lines of L4 L2
  measures "d150" distance between parallel lines of L5 L0
extrude "押し出し10" cut sketch "スケッチ10" against normal blind 3
sketch "スケッチ11" plane through (0, 0, 3) normal (0, 0, 1) x (1, 0, 0)
  circle A0 centre (65, 58.3987) radius 2.25
  circle A1 centre (65, 131.8987) radius 2.25
  line L0 (42.2196, 48.3987) -> (75, 48.3987) construction
  line L1 (75, 48.3987) -> (75, 215) construction
  line L2 (75, 48.3987) -> (75, 215) construction
  circle A2 centre (52.1306, 126.1487) radius 1.2 construction
  circle A3 centre (52.1306, 137.6487) radius 1.2 construction
  line L3 (52.1306, 126.1487) -> (65, 131.8987) construction
  circle A4 centre (52.1306, 137.6487) radius 1.2 construction
  line L4 (65, 131.8987) -> (52.1306, 137.6487) construction
  line L5 (-55, 220) -> (-24.5, 220)
  line L6 (-24.5, 220) -> (-24.5, 232.5)
  line L7 (-24.5, 232.5) -> (-55, 232.5)
  line L8 (-55, 232.5) -> (-55, 220)
  line L9 (55, 220) -> (24.5, 220)
  line L10 (24.5, 220) -> (24.5, 232.5)
  line L11 (24.5, 232.5) -> (55, 232.5)
  line L12 (55, 232.5) -> (55, 220)
  line L13 (70, 184.5) -> (57.5, 184.5)
  line L14 (-55, -220) -> (-24.5, -220)
  line L15 (-24.5, -220) -> (-24.5, -232.5)
  line L16 (-24.5, -232.5) -> (-55, -232.5)
  line L17 (-55, -232.5) -> (-55, -220)
  line L18 (-55, -232.5) -> (55, -232.5) projected
  line L19 (55, -220) -> (24.5, -220)
  line L20 (24.5, -220) -> (24.5, -232.5)
  line L21 (24.5, -232.5) -> (55, -232.5)
  line L22 (55, -232.5) -> (55, -220)
  circle A5 centre (17, 225) radius 2.25
  circle A6 centre (-17, 225) radius 2.25
  circle A7 centre (65, 174.5) radius 2.25
  circle A8 centre (17, -225) radius 2.25
  circle A9 centre (-17, -225) radius 2.25
  line L23 (-55, 232.5) -> (-55, 215) projected
  line L24 (55, 215) -> (55, 232.5) projected
  line L25 (55, 232.5) -> (-55, 232.5) projected
  line L26 (57.5, 184.5) -> (57.5, 215)
  line L27 (57.5, 215) -> (70, 215)
  line L28 (70, 215) -> (70, 184.5)
  line L29 (75, 215) -> (55, 215) projected
  line L30 (-55, -215) -> (-55, -232.5) projected
  line L31 (55, -232.5) -> (55, -215) projected
  point P0 (0, 0)
  point P1 (75, 220.7754)
  dimension "d115" = 10
  dimension "d116" = 10
  dimension "d117" = 4.5
  dimension "d118" = 10
  dimension "d119" = 4.5
  dimension "d120" = 30.5
  dimension "d121" = 10
  dimension "d122" = 10
  dimension "d125" = 7.5
  dimension "d126" = 7.5
  dimension "d127" = 7.5
  dimension "d128" = 7.5
  dimension "d129" = 7.5
  dimension "d130" = 7.5
  dimension "d133" = 12.5
  dimension "d134" = 7.5
  dimension "d135" = 7.5
  dimension "d136" = 2.5
  dimension "d170" = 5
  constraints: 44 end point, 10 point on line, 9 equal length, 8 parallel, 7 centre point, 5 equal radius, 5 horizontal, 5 perpendicular, 2 vertical
  measures "d115" distance from line of A0.centre L0
  measures "d116" distance from line of L1 A0.centre
  measures "d117" diameter of A0
  measures "d118" distance from line of L2 L3.end
  measures "d119" diameter of A1
  measures "d120" distance between parallel lines of L8 L6
  measures "d121" distance from line of A7.centre L1
  measures "d122" distance from line of L13 A7.centre
  measures "d125" distance from line of A5.centre L10
  measures "d126" distance from line of L6 A6.centre
  measures "d127" distance from line of A8.centre L20
  measures "d128" distance from line of L15 A9.centre
  measures "d129" distance from line of L18 A8.centre
  measures "d130" distance from line of L18 A9.centre
  measures "d133" distance of L5.end L6.end
  measures "d134" distance from line of L25 A6.centre
  measures "d135" distance from line of L25 A5.centre
  measures "d136" distance from line of L12 L26.end
  measures "d170" distance from line of L23.end L5
extrude "押し出し11" cut sketch "スケッチ11" against normal blind 3
sketch "スケッチ12" plane through (0, 0, 0) normal (0, 0, -1) x (-1, 0, 0)
  line L0 (-75, 215) -> (-70, 215) projected
  line L1 (-70, 184.5) -> (-75, 184.5)
  line L2 (-75, 184.5) -> (-75, 215)
  line L3 (-75, 215) -> (-70, 215)
  line L4 (-70, 215) -> (-70, 184.5)
  point P0 (0, 0)
  constraints: 8 end point, 2 parallel, 1 horizontal, 1 perpendicular
extrude "押し出し12" cut sketch "スケッチ12" against normal blind 3
sketch "スケッチ13" plane through (0, 0, 0) normal (0, 0, -1) x (-1, 0, 0)
  line L0 (-42.2196, -115.1237) -> (-75, -115.1237) projected
  line L1 (-75, -115.1237) -> (-59, -115.1237)
  line L2 (-59, -115.1237) -> (-59, -110.1237)
  line L3 (-59, -110.1237) -> (-75, -110.1237)
  line L4 (-75, -110.1237) -> (-75, -115.1237)
  point P0 (0, 0)
  dimension "d139" = 16
  dimension "d140" = 5
  constraints: 8 end point, 2 parallel, 1 horizontal, 1 perpendicular
  measures "d139" distance of L3.end L2.end
  measures "d140" distance of L2.end L1.end
extrude "押し出し13" add sketch "スケッチ13" against normal blind 3
sketch "スケッチ14" plane through (0, 0, 0) normal (0, 0, -1) x (-1, 0, 0)
  circle A0 centre (-65, -117.6237) radius 2.25
  line L0 (-75, -110.1237) -> (-75, -215) projected
  line L1 (-59, -110.1237) -> (-75, -110.1237) projected
  line L2 (-59, -115.1237) -> (-42.2196, -115.1237) projected
  line L3 (-59, -115.1237) -> (-64, -110.1237)
  line L4 (-75, -110.1237) -> (-59, -110.1237) projected
  line L5 (-59, -115.1237) -> (-59, -110.1237) projected
  point P0 (0, 0)
  dimension "d143" = 4.5
  dimension "d144" = 10
  dimension "d145" = 7.5
  dimension "d146" = 45
  constraints: 2 end point, 1 centre point, 1 point on line
  measures "d143" diameter of A0
  measures "d144" distance from line of L0 A0.centre
  measures "d145" distance from line of L1 A0.centre
  measures "d146" angle of L5 L3
extrude "押し出し14" cut sketch "スケッチ14" against normal blind 3
sketch "スケッチ15" plane through (0, 0, 3) normal (0, 0, 1) x (1, 0, 0)
  line L0 (40.7196, 49.7705) -> (42.2196, 49.7705) construction
  line L1 (41.4696, 49.7705) -> (41.4696, 47.3672) construction
  arc A0 (43.8196, 48.2705) -> (39.1196, 48.2705) centre (41.4696, 47.3672) ccw
  line L2 (39.1196, 48.2705) -> (43.8196, 48.2705)
  line L3 (42.2196, 48.3987) -> (75, 48.3987) projected
  line L4 (40.7196, 42.2705) -> (40.7196, 27.7705) projected
  line L5 (40.7196, -95.2295) -> (40.7196, -80.7295) projected
  line L6 (40.7196, 42.2705) -> (40.7196, -95.2295) construction
  line L7 (40.7196, -26.4795) -> (52.4195, -26.4795) construction
  line L8 (40.7196, -102.7295) -> (42.2196, -102.7295) construction
  arc A1 (39.1196, -101.2295) -> (43.8196, -101.2295) centre (41.4696, -100.3262) ccw
  line L9 (39.1196, -101.2295) -> (43.8196, -101.2295)
  point P0 (0, 0)
  point P1 (41.4696, -102.7295)
  point P2 (42.2196, -101.3578)
  dimension "d156" = 137.5
  dimension "d157" = 68.75
  constraints: 12 end point, 7 symmetric about line, 6 point on circle, 2 centre point, 2 coincident, 2 midpoint, 2 vertical, 1 horizontal, 1 parallel, 1 other
  measures "d156" distance of L4.start L5.start
  measures "d157" distance from line of L7 L4.start
extrude "押し出し15" cut sketch "スケッチ15" against normal through all
sketch "スケッチ16" plane through (0, 0, 3) normal (0, 0, 1) x (1, 0, 0)
  arc A0 (43.7662, 48.3987) -> (39.1196, 48.2705) centre (41.4696, 47.3672) ccw construction
  line L0 (39.1196, 48.2705) -> (40.7196, 48.2705)
  line L1 (40.7196, 48.2705) -> (40.7196, 49.7705)
  arc A1 (43.7662, 48.3987) -> (39.1196, 48.2705) centre (41.4696, 47.3672) ccw projected
  line L2 (40.7196, 27.7705) -> (40.7196, 42.2705) projected
  line L3 (39.1196, 42.2705) -> (39.1196, 48.2705) projected
  arc A2 (40.7196, 49.7705) -> (39.1196, 48.2705) centre (41.4696, 47.3672) ccw
  line L4 (39.1196, 45.2705) -> (41.0089, 45.2705) construction
  line L5 (39.1196, 42.2705) -> (40.7196, 42.2705)
  line L6 (40.7196, 42.2705) -> (40.7196, 40.7705)
  arc A3 (39.1196, 42.2705) -> (40.7196, 40.7705) centre (41.4696, 43.1738) ccw
  line L7 (39.1196, 27.7705) -> (40.7196, 27.7705)
  line L8 (40.7196, 27.7705) -> (40.7196, 29.2705)
  arc A4 (40.7196, 29.2705) -> (39.1196, 27.7705) centre (41.4696, 26.8672) ccw
  line L9 (39.1196, 24.7705) -> (41.0089, 24.7705) construction
  line L10 (39.1196, 21.7705) -> (40.7196, 21.7705)
  line L11 (40.7196, 21.7705) -> (40.7196, 20.2705)
  arc A5 (39.1196, 21.7705) -> (40.7196, 20.2705) centre (41.4696, 22.6738) ccw
  line L12 (39.1196, 7.2705) -> (40.7196, 7.2705)
  line L13 (40.7196, 7.2705) -> (40.7196, 8.7705)
  arc A6 (40.7196, 8.7705) -> (39.1196, 7.2705) centre (41.4696, 6.3672) ccw
  line L14 (39.1196, 4.2705) -> (41.0089, 4.2705) construction
  line L15 (39.1196, 1.2705) -> (40.7196, 1.2705)
  line L16 (40.7196, 1.2705) -> (40.7196, -0.2295)
  arc A7 (39.1196, 1.2705) -> (40.7196, -0.2295) centre (41.4696, 2.1738) ccw
  line L17 (39.1196, -13.2295) -> (40.7196, -13.2295)
  line L18 (40.7196, -13.2295) -> (40.7196, -11.7295)
  arc A8 (40.7196, -11.7295) -> (39.1196, -13.2295) centre (41.4696, -14.1328) ccw
  line L19 (39.1196, -16.2295) -> (41.0089, -16.2295) construction
  line L20 (39.1196, -19.2295) -> (40.7196, -19.2295)
  line L21 (40.7196, -19.2295) -> (40.7196, -20.7295)
  arc A9 (39.1196, -19.2295) -> (40.7196, -20.7295) centre (41.4696, -18.3262) ccw
  line L22 (39.1196, -33.7295) -> (40.7196, -33.7295)
  line L23 (40.7196, -33.7295) -> (40.7196, -32.2295)
  arc A10 (40.7196, -32.2295) -> (39.1196, -33.7295) centre (41.4696, -34.6328) ccw
  line L24 (39.1196, -36.7295) -> (41.0089, -36.7295) construction
  line L25 (39.1196, -39.7295) -> (40.7196, -39.7295)
  line L26 (40.7196, -39.7295) -> (40.7196, -41.2295)
  arc A11 (39.1196, -39.7295) -> (40.7196, -41.2295) centre (41.4696, -38.8262) ccw
  line L27 (39.1196, -54.2295) -> (40.7196, -54.2295)
  line L28 (40.7196, -54.2295) -> (40.7196, -52.7295)
  arc A12 (40.7196, -52.7295) -> (39.1196, -54.2295) centre (41.4696, -55.1328) ccw
  line L29 (39.1196, -57.2295) -> (41.0089, -57.2295) construction
  line L30 (39.1196, -60.2295) -> (40.7196, -60.2295)
  line L31 (40.7196, -60.2295) -> (40.7196, -61.7295)
  arc A13 (39.1196, -60.2295) -> (40.7196, -61.7295) centre (41.4696, -59.3262) ccw
  line L32 (39.1196, -74.7295) -> (40.7196, -74.7295)
  line L33 (40.7196, -74.7295) -> (40.7196, -73.2295)
  arc A14 (40.7196, -73.2295) -> (39.1196, -74.7295) centre (41.4696, -75.6328) ccw
  line L34 (39.1196, -77.7295) -> (41.0089, -77.7295) construction
  line L35 (39.1196, -80.7295) -> (40.7196, -80.7295)
  line L36 (40.7196, -80.7295) -> (40.7196, -82.2295)
  arc A15 (39.1196, -80.7295) -> (40.7196, -82.2295) centre (41.4696, -79.8262) ccw
  line L37 (39.1196, -95.2295) -> (40.7196, -95.2295)
  line L38 (40.7196, -95.2295) -> (40.7196, -93.7295)
  arc A16 (40.7196, -93.7295) -> (39.1196, -95.2295) centre (41.4696, -96.1328) ccw
  line L39 (39.1196, -98.2295) -> (41.0089, -98.2295) construction
  line L40 (39.1196, -101.2295) -> (40.7196, -101.2295)
  line L41 (40.7196, -101.2295) -> (40.7196, -102.7295)
  arc A17 (39.1196, -101.2295) -> (40.7196, -102.7295) centre (41.4696, -100.3262) ccw
  point P0 (0, 0)
  dimension "d165" = 20.5
  constraints: 80 end point, 33 point on circle, 16 centre point, 16 coincident, 4 symmetric about line, 2 horizontal, 1 midpoint, 1 perpendicular, 1 point on line, 1 vertical, 148 other
  measures "d165" distance of L0.start L7.start
extrude "押し出し16" cut sketch "スケッチ16" against normal through all contours L7 A4 L2 | A3 L5 L2 | L10 L11 A5 | A6 L13 L12 | L15 L16 A7 | A8 L18 L17 | L20 L21 A9 | A10 L23 L22 | L25 L26 A11 | A12 L28 L27 | L30 L31 A13 | A14 L33 L32 | L35 L36 A15 | A16 L38 L37
fillet "フィレット4" radius 2 32 edges at (43.7662, 48.3987, 1.5) (40.7196, 40.7705, 1.5) (40.7196, 29.2705, 1.5) (40.7196, 20.2705, 1.5) (40.7196, 8.7705, 1.5) (40.7196, -0.2295, 1.5) (40.7196, -11.7295, 1.5) (40.7196, -20.7295, 1.5) (40.7196, -32.2295, 1.5) (40.7196, -52.7295, 1.5) (40.7196, -61.7295, 1.5) (40.7196, -73.2295, 1.5) (40.7196, -82.2295, 1.5) (40.7196, -93.7295, 1.5) (42.2196, -102.7295, 1.5) (39.1196, -101.2295, 1.5) (39.1196, -95.2295, 1.5) (39.1196, -80.7295, 1.5) (39.1196, -74.7295, 1.5) (39.1196, -60.2295, 1.5) (39.1196, -54.2295, 1.5) (40.7196, -41.2295, 1.5) (39.1196, -39.7295, 1.5) (39.1196, -33.7295, 1.5) (39.1196, -19.2295, 1.5) (39.1196, -13.2295, 1.5) (39.1196, 1.2705, 1.5) (39.1196, 7.2705, 1.5) (39.1196, 27.7705, 1.5) (39.1196, 21.7705, 1.5) (39.1196, 42.2705, 1.5) (39.1196, 48.2705, 1.5)
sketch "スケッチ17" plane through (0, 0, 3) normal (0, 0, 1) x (1, 0, 0)
  line L0 (35.0196, -111.4331) -> (34.7396, -111.4331) projected
  line L1 (35.0196, -101.9031) -> (35.0196, -111.4331) projected
  line L2 (34.7396, -101.9031) -> (35.0196, -101.9031) projected
  line L3 (35.0196, -91.0877) -> (34.7396, -91.0877) projected
  line L4 (35.0196, -81.5577) -> (35.0196, -91.0877) projected
  line L5 (34.7396, -81.5577) -> (35.0196, -81.5577) projected
  line L6 (35.0196, -70.7423) -> (34.7396, -70.7423) projected
  line L7 (35.0196, -61.2123) -> (35.0196, -70.7423) projected
  line L8 (34.7396, -61.2123) -> (35.0196, -61.2123) projected
  line L9 (35.0196, -50.3969) -> (34.7396, -50.3969) projected
  line L10 (35.0196, -40.8669) -> (35.0196, -50.3969) projected
  line L11 (34.7396, -40.8669) -> (35.0196, -40.8669) projected
  line L12 (35.0196, -30.0515) -> (34.7396, -30.0515) projected
  line L13 (35.0196, -20.5215) -> (35.0196, -30.0515) projected
  line L14 (34.7396, -20.5215) -> (35.0196, -20.5215) projected
  line L15 (35.0196, -9.7061) -> (34.7396, -9.7061) projected
  line L16 (35.0196, -0.1761) -> (35.0196, -9.7061) projected
  line L17 (34.7396, -0.1761) -> (35.0196, -0.1761) projected
  line L18 (35.0196, 10.6393) -> (34.7396, 10.6393) projected
  line L19 (35.0196, 20.1693) -> (35.0196, 10.6393) projected
  line L20 (34.7396, 20.1693) -> (35.0196, 20.1693) projected
  line L21 (35.0196, 30.9847) -> (34.7396, 30.9847) projected
  line L22 (35.0196, 40.5147) -> (35.0196, 30.9847) projected
  line L23 (34.7396, 40.5147) -> (35.0196, 40.5147) projected
  line L24 (34.7396, 30.9847) -> (34.7396, 40.5147)
  line L25 (34.7396, 10.6393) -> (35.0196, 10.6393) projected
  line L26 (34.7396, 20.1693) -> (34.7396, 10.6393)
  line L27 (34.7396, -0.1761) -> (34.7396, -9.7061)
  line L28 (34.7396, -20.5215) -> (34.7396, -30.0515)
  line L29 (34.7396, -40.8669) -> (34.7396, -50.3969)
  line L30 (34.7396, -61.2123) -> (34.7396, -70.7423)
  line L31 (34.7396, -81.5577) -> (34.7396, -91.0877)
  line L32 (34.7396, -101.9031) -> (34.7396, -111.4331)
  point P0 (0, 0)
  constraints: 16 end point, 6 perpendicular, 1 collinear, 1 vertical
extrude "押し出し17" add sketch "スケッチ17" against normal up to surface (3 mm away)
fillet "フィレット5" radius 20 16 edges at (-19.6194, 195.9875, 1.5) (-0.9633, 212.1987, 1.5) (33.7245, 212.1987, 1.5) (52.3806, 195.9875, 1.5) (52.3806, 150.81, 1.5) (33.7245, 134.5987, 1.5) (-0.9633, 134.5987, 1.5) (-19.6194, 150.81, 1.5) (-0.9633, 129.1987, 1.5) (33.7245, 129.1987, 1.5) (52.3806, 112.9875, 1.5) (52.3806, 67.81, 1.5) (33.7245, 51.5987, 1.5) (-0.9633, 51.5987, 1.5) (-19.6194, 67.81, 1.5) (-19.6194, 112.9875, 1.5)
fillet "フィレット6" radius 1 4 edges at (-24.6194, 208.0635, 1.5) (-69.3194, 208.0635, 1.5) (-69.3194, 49.0635, 1.5) (-24.6194, 49.0635, 1.5)
sketch "スケッチ18" plane through (0, 0, 3) normal (0, 0, 1) x (1, 0, 0)
  line L0 (-24.5, -232.5) -> (24.5, -232.5) construction
  line L1 (-24.5, -232.5) -> (24.5, -232.5) construction
  line L2 (0, -232.5) -> (0, -132.6) construction
  line L3 (58.5, -132.6) -> (-34.5, -132.6) construction
  line L4 (-78, -215) -> (-78, -124.6) construction
  line L5 (78, -215) -> (78, -124.6)
  line L6 (78, -124.6) -> (73, -124.6)
  line L7 (73, -124.6) -> (73, -215)
  line L8 (73, -215) -> (78, -215)
  point P0 (0, 0)
  dimension "d175" = 5
  constraints: 10 end point, 2 perpendicular, 2 symmetric about line, 1 horizontal, 1 midpoint, 1 point on line, 1 vertical
  measures "d175" distance of L5.end L6.end
extrude "押し出し18" add sketch "スケッチ18" against normal up to surface (3 mm away)
fillet "フィレット7" radius 1 4 edges at (42.2196, -115.1237, 1.5) (59, -115.1237, 1.5) (75, -110.1237, 1.5) (64, -110.1237, 1.5)
equation "\"d7\" = d6"
equation "\"d8\" = d6"
equation "\"d9\" = d6"
equation "\"d12\" = d11"
equation "\"d32\" = d29"
equation "\"d48\" = d49"
equation "\"d52\" = d51"
equation "\"d53\" = d51"
equation "\"d54\" = d49"
equation "\"d56\" = d51"
equation "\"d57\" = d49"
equation "\"d58\" = d51"
equation "\"d59\" = d51"
equation "\"d84\" = d70 + d69"
